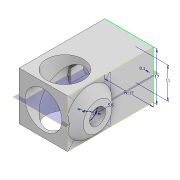
# Autodesk Inventor part: waxing_station
Saved by Autodesk Inventor 2020 (Build 240168000, 168)
## iProperties
Created: 2020-07-20
Part Number: waxing_station
Material: Generic
Document SubType Name: Modeling
Designer: Daniel
Density: 1 g/cm^3
Appearance: Default
Author: Daniel
Autodesk Inventor part; units mm, degrees
ref_plane "YZ Plane" through (0, 0, 0) normal (1, 0, 0) x (0, 1, 0)
ref_plane "XZ Plane" through (0, 0, 0) normal (0, 1, 0) x (-1, 0, 0)
ref_plane "XY Plane" through (0, 0, 0) normal (0, 0, 1) x (1, 0, 0)
sketch "Sketch1" plane through (0, 0, 0) normal (0, 0, 1) x (1, 0, 0)
  line L0 (-8.5, 8.5) -> (8.5, 8.5)
  line L1 (8.5, 8.5) -> (8.5, -8.5)
  line L2 (8.5, -8.5) -> (-8.5, -8.5)
  line L3 (-8.5, -8.5) -> (-8.5, 8.5)
  line L4 (-8.5, 8.5) -> (8.5, -8.5) construction
  line L5 (8.5, 8.5) -> (-8.5, -8.5) construction
  line L6 (5.5, -2.2782) -> (2.2782, -5.5)
  line L7 (2.2782, -5.5) -> (-2.2782, -5.5)
  line L8 (-2.2782, -5.5) -> (-5.5, -2.2782)
  line L9 (-5.5, -2.2782) -> (-5.5, 2.2782)
  line L10 (-5.5, 2.2782) -> (-2.2782, 5.5)
  line L11 (-2.2782, 5.5) -> (2.2782, 5.5)
  line L12 (2.2782, 5.5) -> (5.5, 2.2782)
  line L13 (5.5, 2.2782) -> (5.5, -2.2782)
  line L14 (5.6, -2.3196) -> (2.3196, -5.6)
  line L15 (2.3196, -5.6) -> (-2.3196, -5.6)
  line L16 (-2.3196, -5.6) -> (-5.6, -2.3196)
  line L17 (-5.6, -2.3196) -> (-5.6, 2.3196)
  line L18 (-5.6, 2.3196) -> (-2.3196, 5.6)
  line L19 (-2.3196, 5.6) -> (2.3196, 5.6)
  line L20 (2.3196, 5.6) -> (5.6, 2.3196)
  line L21 (5.6, 2.3196) -> (5.6, -2.3196)
  point P0 (0, 0)
  dimension "d2" = 17
  dimension "d3" = 17
  dimension "d28" = 11
  dimension "d29" = 0.1
  constraints: 44 end point, 2 horizontal, 2 parallel, 1 midpoint, 1 perpendicular, 24 other
  measures "d2" distance of L1.end L2.end
  measures "d3" distance of L0.end L1.end
  measures "d28" distance between parallel lines of L11 L7
  measures "d29" distance between parallel lines of L13 L21
extrude "Extrusion1" add sketch "Sketch1" along normal blind 30 contours L0 L1 L2 L3 | L6 L7 L8 L9 L10 L11 L12 L13 | L14 L15 L16 L17 L18 L19 L20 L21
extrude "Extrusion2" cut sketch "Sketch1" along normal blind 15 contours L6 L7 L8 L9 L10 L11 L12 L13 | L14 L15 L16 L17 L18 L19 L20 L21
sketch "Sketch2" plane through (0, 0, 30) normal (0, 0, 1) x (1, 0, 0)
  circle A0 centre (0, 0) radius 6.425
  dimension "d8" = 12.85
  constraints: 1 centre point, 1 coincident
  measures "d8" diameter of A0
extrude "Extrusion3" cut sketch "Sketch2" against normal blind 15
sketch "Sketch3" plane through (-8.5, 8.5, 0) normal (0, 1, 0) x (1, 0, 0)
  line L0 (17, 0) -> (0, 0) projected
  line L1 (0, 0) -> (0, -30) projected
  line L2 (17, -30) -> (0, -30) projected
  line L3 (17, 0) -> (17, -30) projected
  line L4 (0, 0) -> (0, -30) construction
  line L5 (0, -30) -> (17, -15)
  line L6 (17, 0) -> (17, -30) construction
  circle A0 centre (8.5, -22.5) radius 6.425
  line L7 (17, -30) -> (0, -15)
  line L8 (0, 0) -> (0, -30) construction
  point P0 (8.5, 0)
  dimension "d11" = 12.85
  constraints: 4 end point, 3 midpoint, 1 centre point
  measures "d11" diameter of A0
extrude "Extrusion4" cut sketch "Sketch3" against normal through all contours A0 L7 L5 | L5 L7 A0 | L7 L5 A0 | A0 L5 L7
sketch "Sketch4" plane through (8.5, -8.5, 0) normal (1, 0, 0) x (0, 0, -1)
  line L0 (0, 17) -> (-30, 17) construction
  line L1 (-15, 17) -> (-15, 0) construction
  line L2 (0, 0) -> (-30, 0) construction
  line L3 (-30, 17) -> (-30, 0) construction
  line L4 (-30, 17) -> (-15, 0) construction
  line L5 (-15, 17) -> (-30, 0) construction
  circle A0 centre (-22.5, 8.5) radius 2.8
  circle A1 centre (-22.5, 8.5) radius 5
  point P0 (0, 8.5)
  dimension "d14" = 5.6
  dimension "d15" = 10
  constraints: 6 end point, 3 midpoint, 2 centre point, 1 coincident
  measures "d14" diameter of A0
  measures "d15" diameter of A1
ref_plane "Work Plane1" through (-8.5, 0, 0) normal (0, -1, 0) x (1, 0, 0)
sketch "Sketch5" plane through (-8.5, 0, 0) normal (0, -1, 0) x (1, 0, 0)
  line L0 (17, 0) -> (17, 30) construction
  line L1 (0, 0) -> (0, 30) construction
  line L2 (17, 0) -> (0, 0) construction
  line L3 (17, 30) -> (0, 30) construction
  point P0 (8.5, 0)
  point P1 (17, 22.5)
  point P2 (0, 7.5)
  dimension "d23" = 7.5
  dimension "d24" = 7.5
  constraints: 2 point on line
  measures "d23" distance from line of L2 point (0, 7.5)
  measures "d24" distance from line of L3 point (17, 22.5)
extrude "Extrusion5" add sketch "Sketch4" along normal blind 3
extrude "Extrusion6" cut sketch "Sketch4" against normal blind 5 contours A0
pattern_sketch "Sketch Driven Pattern1" of "Extrusion6", "Extrusion5" from (8.5, 0, 22.5) facing (1, 0, 0) copies at (-8.5, 0, 7.5) facing (-1, 0, 0)
chamfer "Chamfer2" distance 3 angle 45 2 edges at (8.5, 0, 27.5) (-8.5, 0, 2.5)
equation "\"d2\" = d3"
equation "\"d23\" = d24"
body "Solid1"
